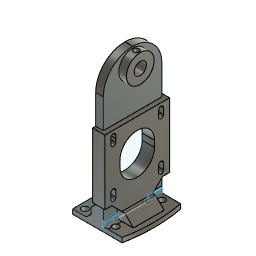
Right handle (Autodesk Fusion 360 design; units mm, degrees)
Autodesk Fusion 360 part; units mm, degrees
note: some values were not read from the file. Set by a fixed rule: which face or edge a step refers to.
sketch "Szkic1" plane through (0, 0, 0) normal (0, 0, 1) x (1, 0, 0)
  circle A0 centre (0, 0) radius 100
  line L0 (66, 19) -> (66, -19)
  line L1 (66, -19) -> (98.1784, -19)
  line L2 (66, 19) -> (98.1784, 19)
  dimension "d1" = 200
  constraint coincident A0.centre origin
  constraint coincident A0 L1.end
  constraint perpendicular L0 L1
  constraint coincident A0 L2.end
  constraint perpendicular L0 L2
  measures "d1" diameter of A0
extrude "Wyciągnięcie proste1" add sketch "Szkic1" along normal blind 3 contours A0 L0 L1 L2 picked at (77.3333, 0)
move_face "Przesuń powierzchnię1" by (-33, 0, 0) 1 faces at (77.3333, 0, 3)
move_body "Przesuń1" bodies 1 to x (1, 0, 0) y (0, 1, 0) z (0, 0, 1) at (-66, 0, 0)
sketch "Szkic2" plane through (0, 0, 3) normal (0, 0, 1) x (-1, 0, 0)
  line L0 (0, 19) -> (-32.1784, 19)
  arc A0 (-32.1784, 19) -> (-32.1784, -19) centre (66, 0) ccw
  line L1 (-32.1784, -19) -> (0, -19)
  line L2 (0, -19) -> (0, 19)
  circle A1 centre (-4, -15) radius 2.1
  circle A2 centre (-24, -15) radius 2.1
  circle A3 centre (-4, 15) radius 2.1
  circle A4 centre (-24, 15) radius 2.1
  dimension "d5" = 4.2
  dimension "d6" = 4.2
  dimension "d7" = 4.2
  dimension "d8" = 4.2
  measures "d5" diameter of A1
  measures "d6" diameter of A2
  measures "d7" diameter of A3
  measures "d8" diameter of A4
extrude "Wyciągnięcie proste2" cut sketch "Szkic2" against normal blind 3 contours A1 | A2 | A3 | A4
sketch "Szkic3" plane through (0, 0, 3) normal (0, 0, 1) x (-1, 0, 0)
  circle A0 centre (-4, 15) radius 2.1
  circle A1 centre (-24, 15) radius 2.1
  circle A2 centre (-4, -15) radius 2.1
  circle A3 centre (-24, -15) radius 2.1
  line L0 (0, 19) -> (-32.1784, 19)
  arc A4 (-32.1784, 19) -> (-32.1784, -19) centre (66, 0) ccw
  line L1 (-32.1784, -19) -> (0, -19)
  line L2 (0, -19) -> (0, 19)
  line L3 (-15, -19) -> (-20, -19)
  line L4 (-20, -19) -> (-20, 19)
  line L5 (-20, 19) -> (-15, 19)
  line L6 (-15, 19) -> (-15, -19)
  constraint horizontal L3
  constraint vertical L4
  constraint horizontal L5
  constraint vertical L6
  constraint coincident L0 L4.end
  constraint coincident L1 L3.start
extrude "Wyciągnięcie proste3" add sketch "Szkic3" along normal blind 72 contours L0 L1 L3 L4 L5 L6
extrude "Wyciągnięcie proste4" add 1 faces at (18.3333, -6.3333, 75) along direction (0, 0, 1) blind 30
extrude "Wyciągnięcie proste5" cut 1 faces at (18.3333, -6.3333, 105) along direction (0, 0, -1) blind 10
sketch "Szkic4" plane through (15, 0, 0) normal (-1, 0, 0) x (0, -1, 0)
  line L0 (19, 95) -> (-19, 95)
  line L1 (-19, 95) -> (-19, 3)
  line L2 (-19, 3) -> (19, 3)
  line L3 (19, 3) -> (19, 95)
  circle A0 centre (0, 85) radius 4
extrude "Wyciągnięcie proste6" cut sketch "Szkic4" against normal blind 5 contours A0
fillet "Zaokrąglenie1" radius 19 2 edges at (17.5, -19, 95) (17.5, 19, 95)
sketch "Szkic5" plane through (20, 0, 0) normal (1, 0, 0) x (0, 1, 0)
  circle A0 centre (0, 85) radius 4
  arc A1 (19, 76) -> (0, 95) centre (0, 76) ccw
  arc A2 (0, 95) -> (-19, 76) centre (0, 76) ccw
  line L0 (-19, 76) -> (-19, 3)
  line L1 (-19, 3) -> (19, 3)
  line L2 (19, 3) -> (19, 76)
  circle A3 centre (0, 85) radius 9
  dimension "d21" = 18
  constraint concentric A0 A3
  measures "d21" diameter of A3
extrude "Wyciągnięcie proste7" add sketch "Szkic5" along normal blind 5 contours A3
sketch "Szkic6" plane through (0, 0, 3) normal (0, 0, 1) x (-1, 0, 0)
  line L0 (-20, -19) -> (-20, 19)
  line L1 (-20, 19) -> (-32.1784, 19)
  arc A0 (-32.1784, 19) -> (-32.1784, -19) centre (66, 0) ccw
  line L2 (-32.1784, -19) -> (-20, -19)
  circle A1 centre (-24, -15) radius 2.1
  circle A2 centre (-24, 15) radius 2.1
  circle A3 through (-20.7, 0, 92.5) (-23.4, 1.5588, 92.5) (-23.4, -1.5588, 92.5)
  dimension "d24" = 3.6
extrude "Wyciągnięcie proste8" cut sketch "Szkic6" against normal blind 8 contours A3 in plane through (0, 0, 95.5) normal (0, 0, 1)
sketch "Szkic7" plane through (0, 0, 0) normal (0, 1, 0) x (1, 0, 0)
  line L0 (20, -35) -> (28, -35)
  line L1 (28, -35) -> (28, -3)
  line L2 (28, -3) -> (20, -3)
  line L3 (20, -3) -> (20, -35)
  line L4 (15, -35) -> (7, -35)
  line L5 (7, -35) -> (7, -3)
  line L6 (7, -3) -> (15, -3)
  line L7 (15, -3) -> (15, -35)
  constraint horizontal L0
  constraint vertical L1
  constraint horizontal L2
  constraint vertical L3
  constraint horizontal L4
  constraint vertical L5
  constraint horizontal L6
  constraint vertical L7
extrude "Wyciągnięcie proste9" add sketch "Szkic7" along normal mid plane 16
extrude "Wyciągnięcie proste10" cut 2 faces at (25.3333, 2.6667, 35) (9.6667, 2.6667, 35) along direction (0, 0, -1) blind 28
sketch "Szkic8" plane through (20, 0, 0) normal (1, 0, 0) x (0, 1, 0)
  line L0 (8, 7) -> (8, 3)
  line L1 (8, 3) -> (19, 3)
  line L2 (19, 3) -> (19, 76)
  arc A0 (19, 76) -> (0, 95) centre (0, 76) ccw
  arc A1 (0, 95) -> (-19, 76) centre (0, 76) ccw
  line L3 (-19, 76) -> (-19, 3)
  line L4 (-19, 3) -> (-8, 3)
  line L5 (-8, 3) -> (-8, 7)
  line L6 (-8, 7) -> (8, 7)
  circle A2 centre (0, 85) radius 9
  line L7 (-8, 7) -> (8, 7)
  line L8 (8, 7) -> (8, 35)
  line L9 (8, 35) -> (-8, 35)
  line L10 (-8, 35) -> (-8, 7)
  constraint horizontal L7
  constraint vertical L8
  constraint horizontal L9
  constraint vertical L10
  constraint coincident L5.end L6.start
extrude "Wyciągnięcie proste11" add sketch "Szkic8" along normal blind 4 and the other way blind 9 contours L6 L7 L8 L9 L10
extrude "Wyciągnięcie proste12" cut 1 faces at (11, 2.6667, 25.6667) along direction (1, 0, 0) blind 1
extrude "Wyciągnięcie proste13" cut 2 faces at (11.3333, -2.6667, 7) (9.6667, -2.6667, 7) along direction (0, 0, -1) blind 2
extrude "Wyciągnięcie proste14" add 2 faces at (14, -8, 5) (13, -8, 25.6667) along direction (0, -1, 0) blind 11
extrude "Wyciągnięcie proste15" add 2 faces at (14, 8, 5) (13, 8, 25.6667) along direction (0, 1, 0) blind 11
extrude "Wyciągnięcie proste16" cut 1 faces at (10.3333, -6.3333, 5) along direction (0, 0, -1) blind 2
extrude "Wyciągnięcie proste17" cut 1 faces at (12, -6.3333, 15) along direction (1, 0, 0) blind 3
fillet "Zaokrąglenie2" radius 6 1 edges at (15, 0, 3)
extrude "Wyciągnięcie proste18" cut 1 faces at (22.6667, 2.6667, 35) along direction (0, 0, -1) blind 20
extrude "Wyciągnięcie proste19" add 1 faces at (28, 2.6667, 5.6667) along direction (1, 0, 0) blind 3
sketch "Szkic9" plane through (15, 0, 0) normal (-1, 0, 0) x (0, -1, 0)
  circle A0 centre (0, 85) radius 4
  line L0 (-19, 9) -> (19, 9)
  line L1 (19, 9) -> (19, 76)
  arc A1 (19, 76) -> (0, 95) centre (0, 76) ccw
  arc A2 (0, 95) -> (-19, 76) centre (0, 76) ccw
  line L2 (-19, 76) -> (-19, 9)
  line L3 (0, 85) -> (0, 36)
  line L4 (15.5, 20.5) -> (-15.5, 51.5) construction
  line L5 (-15.5, 20.5) -> (15.5, 51.5) construction
  circle A3 centre (-15.5, 51.5) radius 1.6
  circle A4 centre (15.5, 51.5) radius 1.6
  circle A5 centre (15.5, 20.5) radius 1.6
  circle A6 centre (-15.5, 20.5) radius 1.6
  point P0 (0, 36)
  dimension "d53" = 31
  dimension "d54" = 31
  dimension "d55" = 3.2
  dimension "d56" = 3.2
  dimension "d57" = 3.2
  dimension "d58" = 3.2
  constraint coincident A0.centre L3.start
  constraint vertical L3
  constraint coincident L4 P0
  constraint coincident L5 P0
  constraint coincident P0 L3.end
  constraint coincident L4.end A3.centre
  constraint coincident L5.end A4.centre
  constraint coincident L4.start A5.centre
  constraint coincident L5.start A6.centre
  measures "d53" distance of L4.end L5.end
  measures "d54" distance of L5.start L4.end
  measures "d55" diameter of A3
  measures "d56" diameter of A4
  measures "d57" diameter of A5
  measures "d58" diameter of A6
extrude "Wyciągnięcie proste20" cut sketch "Szkic9" against normal blind 5 contours A3 | A4 | A5 | A6
sketch "Szkic10" plane through (0, -19, 0) normal (0, -1, 0) x (1, 0, 0)
  arc A0 (9, 3) -> (15, 9) centre (9, 9) ccw
  line L0 (9, 3) -> (0, 3)
  line L1 (0, 3) -> (0, 0)
  line L2 (0, 0) -> (32.1784, 0)
  line L3 (32.1784, 0) -> (32.1784, 3)
  line L4 (32.1784, 3) -> (20, 3)
  line L5 (20, 3) -> (20, 76)
  line L6 (20, 76) -> (15, 76)
  line L7 (15, 76) -> (15, 9)
sketch "Szkic11" plane through (15, 0, 0) normal (-1, 0, 0) x (0, -1, 0)
  circle A0 centre (-15.5, 51.5) radius 1.6
  circle A1 centre (15.5, 51.5) radius 1.6
  circle A2 centre (-15.5, 20.5) radius 1.6
  circle A3 centre (15.5, 20.5) radius 1.6
  circle A4 centre (0, 85) radius 4
  line L0 (-19, 9) -> (19, 9)
  line L1 (19, 9) -> (19, 76)
  arc A5 (19, 76) -> (0, 95) centre (0, 76) ccw
  arc A6 (0, 95) -> (-19, 76) centre (0, 76) ccw
  line L2 (-19, 76) -> (-19, 9)
  line L3 (-15.5, 51.5) -> (15.5, 51.5)
  line L4 (15.5, 51.5) -> (15.5, 20.5)
  line L5 (15.5, 20.5) -> (-15.5, 20.5)
  line L6 (-15.5, 20.5) -> (-15.5, 51.5)
  line L7 (21, 17) -> (-21, 17)
  line L8 (-21, 17) -> (-21, 55)
  line L9 (-21, 55) -> (21, 55)
  line L10 (21, 55) -> (21, 17)
  line L11 (21, 17) -> (-21, 55) construction
  line L12 (-21, 17) -> (21, 55) construction
  line L13 (-19, 55) -> (19, 55)
  line L14 (19, 55) -> (19, 17)
  line L15 (19, 17) -> (-19, 17)
  line L16 (-19, 17) -> (-19, 55)
  point P0 (0, 36)
  dimension "d61" = 42
  constraint horizontal L3
  constraint vertical L4
  constraint horizontal L5
  constraint vertical L6
  constraint coincident A3.centre L4.end
  constraint coincident A0.centre L3.start
  constraint horizontal L7
  constraint perpendicular L7 L8
  constraint parallel L7 L9
  constraint parallel L8 L10
  constraint coincident L11 P0
  constraint coincident L12 P0
  constraint horizontal L13
  constraint vertical L14
  constraint horizontal L15
  constraint vertical L16
  constraint coincident L1 L14.end
  constraint coincident L7 L14.end
  constraint coincident L9 L13.start
  constraint coincident L2 L13.start
  measures "d61" distance of L8.end L9.end
extrude "Wyciągnięcie proste21" add sketch "Szkic11" against normal blind 5 contours L2 L7 L8 L9 L16 | L1 L7 L9 L10 L14
extrude "Wyciągnięcie proste22" cut 1 faces at (22.6667, 2.6667, 15) along direction (0, 0, -1) blind 12
extrude "Wyciągnięcie proste23" cut 1 faces at (31, 2.6667, 5.6667) along direction (-1, 0, 0) blind 9
delete_face "Usuń powierzchnię1" 1 faces at (9.5703, -6.3333, 3.0272)
sketch "Szkic12" plane through (15, 0, 0) normal (-1, 0, 0) x (0, -1, 0)
  circle A0 centre (0, 85) radius 4
  circle A1 centre (15.5, 20.5) radius 1.6
  circle A2 centre (-15.5, 20.5) radius 1.6
  circle A3 centre (15.5, 51.5) radius 1.6
  circle A4 centre (-15.5, 51.5) radius 1.6
  line L0 (-19, 3) -> (19, 3)
  line L1 (19, 3) -> (19, 17)
  line L2 (19, 17) -> (21, 17)
  line L3 (21, 17) -> (21, 55)
  line L4 (21, 55) -> (19, 55)
  line L5 (19, 55) -> (19, 76)
  arc A5 (19, 76) -> (0, 95) centre (0, 76) ccw
  arc A6 (0, 95) -> (-19, 76) centre (0, 76) ccw
  line L6 (-19, 76) -> (-19, 55)
  line L7 (-19, 55) -> (-21, 55)
  line L8 (-21, 55) -> (-21, 17)
  line L9 (-21, 17) -> (-19, 17)
  line L10 (-19, 17) -> (-19, 3)
  line L11 (-19, 3) -> (19, 3)
  line L12 (19, 3) -> (19, 10)
  line L13 (19, 10) -> (-19, 10)
  line L14 (-19, 10) -> (-19, 3)
  constraint horizontal L11
  constraint vertical L12
  constraint horizontal L13
  constraint vertical L14
  constraint midpoint L1 L12.end
  constraint coincident L0.start L10.end
extrude "Wyciągnięcie proste24" add sketch "Szkic12" along normal blind 3 contours L0 L1 L10 L11 L12 L13 L14
sketch "Szkic13" plane through (0, 0, 3) normal (0, 0, 1) x (-1, 0, 0)
  line L0 (-12, 19) -> (-12, -19)
  line L1 (-12, -19) -> (0, -19)
  line L2 (0, -19) -> (0, 19)
  line L3 (0, 19) -> (-12, 19)
  circle A0 centre (-4, -15) radius 2.1
  circle A1 centre (-4, 15) radius 2.1
chamfer "Fazowanie1" distance 3 angle 45 2 edges at (15, 0, 10) (12, 0, 3)
sketch "Szkic14" plane through (20, 0, 0) normal (1, 0, 0) x (0, 1, 0)
  circle A0 centre (15.5, 51.5) radius 1.6
  circle A1 centre (-15.5, 51.5) radius 1.6
  circle A2 centre (15.5, 20.5) radius 1.6
  circle A3 centre (-15.5, 20.5) radius 1.6
  line L0 (-19, 3) -> (19, 3)
  line L1 (19, 3) -> (19, 17)
  line L2 (19, 17) -> (21, 17)
  line L3 (21, 17) -> (21, 55)
  line L4 (21, 55) -> (19, 55)
  line L5 (19, 55) -> (19, 76)
  arc A4 (19, 76) -> (0, 95) centre (0, 76) ccw
  arc A5 (0, 95) -> (-19, 76) centre (0, 76) ccw
  line L6 (-19, 76) -> (-19, 55)
  line L7 (-19, 55) -> (-21, 55)
  line L8 (-21, 55) -> (-21, 17)
  line L9 (-21, 17) -> (-19, 17)
  line L10 (-19, 17) -> (-19, 3)
  circle A6 centre (0, 85) radius 9
  line L11 (-10.169, 3) -> (9.831, 3)
  constraint coincident L0 L11.start
  constraint coincident L0 L11.end
chamfer "Fazowanie2" distance 3 angle 45 1 edges at (20, 0, 3)
sketch "Szkic15" plane through (20, 0, 0) normal (1, 0, 0) x (0, 1, 0)
  line L0 (-19, 6) -> (-10, 6)
  line L1 (-10, 6) -> (-10, 3)
  line L2 (-10, 3) -> (-19, 3)
  line L3 (-19, 3) -> (-19, 6)
  line L4 (19, 6) -> (10, 6)
  line L5 (10, 6) -> (10, 3)
  line L6 (10, 3) -> (19, 3)
  line L7 (19, 3) -> (19, 6)
  constraint horizontal L0
  constraint vertical L1
  constraint horizontal L2
  constraint vertical L3
  constraint horizontal L4
  constraint vertical L5
  constraint horizontal L6
  constraint vertical L7
sketch "Szkic16" plane through (0, -19, 0) normal (0, -1, 0) x (1, 0, 0)
  line L0 (9, 3) -> (0, 3)
  line L1 (0, 3) -> (0, 0)
  line L2 (0, 0) -> (32.1784, 0)
  line L3 (32.1784, 0) -> (32.1784, 3)
  line L4 (32.1784, 3) -> (23, 3)
  line L5 (23, 3) -> (20, 6)
  line L6 (20, 6) -> (20, 17)
  line L7 (20, 17) -> (15, 17)
  line L8 (15, 17) -> (15, 13)
  line L9 (15, 13) -> (12, 10)
  line L10 (12, 10) -> (12, 6)
  line L11 (12, 6) -> (9, 3)
  line L12 (20, 6) -> (20, 3)
  line L13 (20, 3) -> (23, 3)
  line L14 (20, 6) -> (23, 3)
  constraint coincident L5.end L6.start
  constraint parallel L6 L12
  constraint coincident L4.end L5.start
extrude "Wyciągnięcie proste25" cut sketch "Szkic16" against normal blind 9 contours L5 L12 L13 L14
sketch "Szkic17" plane through (0, 19, 0) normal (0, 1, 0) x (-1, 0, 0)
  line L0 (0, 3) -> (-9, 3)
  line L1 (-9, 3) -> (-12, 6)
  line L2 (-12, 6) -> (-12, 10)
  line L3 (-12, 10) -> (-15, 13)
  line L4 (-15, 13) -> (-15, 17)
  line L5 (-15, 17) -> (-20, 17)
  line L6 (-20, 17) -> (-20, 6)
  line L7 (-20, 6) -> (-23, 3)
  line L8 (-23, 3) -> (-32.1784, 3)
  line L9 (-32.1784, 3) -> (-32.1784, 0)
  line L10 (-32.1784, 0) -> (0, 0)
  line L11 (0, 0) -> (0, 3)
  line L12 (-20, 6) -> (-23, 3)
  line L13 (-20, 3) -> (-23, 3)
  line L14 (-20, 6) -> (-20, 3)
  constraint coincident L6.end L7.start
  constraint coincident L7.end L8.start
  constraint parallel L8 L13
  constraint parallel L6 L14
extrude "Wyciągnięcie proste26" cut sketch "Szkic17" against normal blind 9 contours L7 L12 L13 L14
extrude "Wyciągnięcie proste27" cut 1 faces at (21, 10, 4) along direction (0, -1, 0) blind 20
sketch "Szkic18" plane through (12, 0, 0) normal (-1, 0, 0) x (0, -1, 0)
  line L0 (-19, 6) -> (19, 6)
  line L1 (19, 6) -> (19, 10)
  line L2 (19, 10) -> (-19, 10)
  line L3 (-19, 10) -> (-19, 6)
sketch "Szkic19" plane through (20, 0, 0) normal (1, 0, 0) x (0, 1, 0)
  circle A0 centre (0, 10) radius 1.8
  dimension "d79" = 3.6
  measures "d79" diameter of A0
extrude "Wyciągnięcie proste28" cut sketch "Szkic19" against normal blind 5.5
sketch "Szkic20" plane through (0, 19, 0) normal (0, 1, 0) x (-1, 0, 0)
  line L0 (-20, 3) -> (-32.1784, 3)
  line L1 (-32.1784, 3) -> (-32.1784, 0)
  line L2 (-32.1784, 0) -> (0, 0)
  line L3 (0, 0) -> (0, 3)
  line L4 (0, 3) -> (-9, 3)
  line L5 (-9, 3) -> (-12, 6)
  line L6 (-12, 6) -> (-12, 10)
  line L7 (-12, 10) -> (-15, 13)
  line L8 (-15, 13) -> (-15, 17)
  line L9 (-15, 17) -> (-20, 17)
  line L10 (-20, 17) -> (-20, 6)
  line L11 (-20, 6) -> (-20, 3)
  line L12 (-20, 7) -> (-20, 3)
  line L13 (-20, 3) -> (-24, 3)
  line L14 (-24, 3) -> (-20, 7)
  constraint coincident L10 L12.start
  constraint coincident L0.start L11.end
  constraint coincident L0 L13.end
  constraint parallel L0 L13
extrude "Wyciągnięcie proste29" add sketch "Szkic20" against normal blind 29 contours L0 L10 L11 L12 L13 L14
sketch "Szkic21" plane through (0, 19, 0) normal (0, 1, 0) x (-1, 0, 0)
  line L0 (-24, 3) -> (-32.1784, 3)
  line L1 (-32.1784, 3) -> (-32.1784, 0)
  line L2 (-32.1784, 0) -> (0, 0)
  line L3 (0, 0) -> (0, 3)
  line L4 (0, 3) -> (-9, 3)
  line L5 (-9, 3) -> (-12, 6)
  line L6 (-12, 6) -> (-12, 10)
  line L7 (-12, 10) -> (-15, 13)
  line L8 (-15, 13) -> (-15, 17)
  line L9 (-15, 17) -> (-20, 17)
  line L10 (-20, 17) -> (-20, 7)
  line L11 (-20, 7) -> (-24, 3)
  line L12 (-20, 7) -> (-24, 3)
  line L13 (-20, 3) -> (-20, 7)
  line L14 (-20, 3) -> (-24, 3)
  constraint coincident L10.end L11.start
  constraint coincident L0.start L11.end
  constraint parallel L10 L13
  constraint parallel L0 L14
extrude "Wyciągnięcie proste30" cut sketch "Szkic21" against normal blind 9 contours L11 L12 L13 L14
sketch "Szkic23" plane through (15, 0, 0) normal (-1, 0, 0) x (0, -1, 0)
  circle A0 centre (-15.5, 53.5) radius 1.6
  circle A1 centre (-15.5, 18.5) radius 1.6
  circle A2 centre (-15.5, 22.5) radius 1.6
  circle A3 centre (15.5, 18.5) radius 1.6
  circle A4 centre (15.5, 22.5) radius 1.6
  circle A5 centre (15.5, 53.5) radius 1.6
  circle A6 centre (15.5, 49.5) radius 1.6
  circle A7 centre (-15.5, 49.5) radius 1.6
  line L0 (-13.9003, 53.4712) -> (-13.9003, 49.4712)
  line L1 (-17.1, 49.5) -> (-17.1, 53.5)
  line L2 (-13.9003, 53.4712) -> (-13.9003, 49.4712)
  line L3 (13.9003, 49.4712) -> (13.9, 53.4999)
  line L4 (17.0997, 53.4712) -> (17.1, 49.5001)
  line L5 (17.1, 22.5001) -> (17.1, 18.5)
  line L6 (13.9, 18.5) -> (13.9, 22.5)
  line L7 (-13.9003, 22.5287) -> (-13.9, 18.5001)
  line L8 (-17.1, 18.5001) -> (-17.1, 22.5)
  dimension "d98" = 3.2
  dimension "d99" = 3.2
  dimension "d100" = 3.2
  dimension "d101" = 3.2
  dimension "d102" = 3.2
  dimension "d103" = 3.2
  dimension "d104" = 3.2
  dimension "d105" = 3.2
  constraint coincident A0 L0.start
  constraint coincident A7 L0.end
  constraint vertical L0
  constraint coincident A7 L1.start
  constraint coincident A0 L1.end
  constraint tangent A0 L1
  constraint vertical L1
  constraint coincident A6 L3.start
  constraint coincident A5 L3.end
  constraint tangent A5 L3
  constraint coincident A5 L4.start
  constraint coincident A6 L4.end
  constraint tangent A6 L4
  constraint coincident A4 L5.start
  constraint coincident A3 L5.end
  constraint tangent A3 L5
  constraint coincident A3 L6.start
  constraint coincident A4 L6.end
  constraint tangent A4 L6
  constraint vertical L6
  constraint coincident A2 L7.start
  constraint coincident A1 L7.end
  constraint tangent A1 L7
  constraint coincident A1 L8.start
  constraint coincident A2 L8.end
  constraint tangent A2 L8
  measures "d98" diameter of A0
  measures "d99" diameter of A1
  measures "d100" diameter of A2
  measures "d101" diameter of A3
  measures "d102" diameter of A4
  measures "d103" diameter of A5
  measures "d104" diameter of A6
  measures "d105" diameter of A7
extrude "Wyciągnięcie proste31" cut sketch "Szkic23" against normal blind 5 contours A0 | A0 A7 L0 L1 L2 | A7 | A1 | A1 A2 L7 L8 | A2 | A3 | A3 A4 L5 L6 | A4 | A5 | A6 | A5 A6 L3 L4
extrude "Wyciągnięcie proste32" add 1 faces at (16.6667, -19.6667, 55) along direction (0, 0, 1) blind 2
extrude "Wyciągnięcie proste33" add 1 faces at (16.6667, 20.3333, 55) along direction (0, 0, 1) blind 2
extrude "Wyciągnięcie proste34" add 2 faces at (16.6667, -20.3333, 17) (16.6667, 19.6667, 17) along direction (0, 0, -1) blind 2
sketch "Szkic24" plane through (15, 0, 0) normal (-1, 0, 0) x (0, -1, 0)
  line L0 (17.1, 22.5001) -> (17.1, 18.5)
  arc A0 (13.9, 18.5) -> (17.1, 18.5) centre (15.5, 18.5) ccw
  line L1 (13.9, 18.5) -> (13.9, 22.5)
  arc A1 (17.1, 22.5001) -> (13.9, 22.5) centre (15.5, 22.5) ccw
  line L2 (-13.9001, 20.4798) -> (-13.9, 18.5001)
  arc A2 (-17.1, 18.5001) -> (-13.9, 18.5001) centre (-15.5, 18.5) ccw
  line L3 (-17.1, 18.5001) -> (-17.1, 22.5)
  arc A3 (-13.9003, 22.5287) -> (-17.1, 22.5) centre (-15.5, 22.5) ccw
  line L4 (-13.9003, 22.5287) -> (-13.9001, 20.5204)
  arc A4 (-13.9001, 20.4798) -> (-13.9001, 20.5204) centre (-15.5, 20.5) ccw
  line L5 (-13.9003, 53.4712) -> (-13.9003, 51.5287)
  arc A5 (-13.9003, 51.4713) -> (-13.9003, 51.5287) centre (-15.5, 51.5) ccw
  line L6 (-13.9003, 51.4713) -> (-13.9003, 49.4712)
  arc A6 (-17.1, 49.5) -> (-13.9003, 49.4712) centre (-15.5, 49.5) ccw
  line L7 (-17.1, 49.5) -> (-17.1, 53.5)
  arc A7 (-13.9003, 53.4712) -> (-17.1, 53.5) centre (-15.5, 53.5) ccw
  line L8 (-19, 13) -> (19, 13)
  line L9 (19, 13) -> (19, 15)
  line L10 (19, 15) -> (21, 15)
  line L11 (21, 15) -> (21, 57)
  line L12 (21, 57) -> (19, 57)
  line L13 (19, 57) -> (19, 76)
  arc A8 (19, 76) -> (0, 95) centre (0, 76) ccw
  arc A9 (0, 95) -> (-19, 76) centre (0, 76) ccw
  line L14 (-19, 76) -> (-19, 57)
  line L15 (-19, 57) -> (-21, 57)
  line L16 (-21, 57) -> (-21, 15)
  line L17 (-21, 15) -> (-19, 15)
  line L18 (-19, 15) -> (-19, 13)
  line L19 (13.9001, 51.5202) -> (13.9, 53.4999)
  arc A10 (17.0997, 53.4712) -> (13.9, 53.4999) centre (15.5, 53.5) ccw
  line L20 (17.0997, 53.4712) -> (17.0999, 51.5205)
  arc A11 (17.0999, 51.4797) -> (17.0999, 51.5205) centre (15.5, 51.5) ccw
  line L21 (17.0999, 51.4797) -> (17.1, 49.5001)
  arc A12 (13.9003, 49.4712) -> (17.1, 49.5001) centre (15.5, 49.5) ccw
  line L22 (13.9003, 49.4712) -> (13.9001, 51.4796)
  arc A13 (13.9001, 51.5202) -> (13.9001, 51.4796) centre (15.5, 51.5) ccw
  circle A14 centre (0, 85) radius 4
sketch "Szkic25" plane through (20, 0, 0) normal (1, 0, 0) x (0, 1, 0)
  line L0 (-21, 57) -> (21, 57)
  line L1 (21, 57) -> (21, 15)
  line L2 (21, 15) -> (-21, 15)
  line L3 (-21, 15) -> (-21, 57)
  constraint horizontal L0
  constraint vertical L1
  constraint horizontal L2
  constraint vertical L3
extrude "Wyciągnięcie proste35" add sketch "Szkic25" along normal blind 5
extrude "Wyciągnięcie proste36" cut sketch "Szkic24" against normal blind 10 contours L0 A0 L1 A1 | L2 A2 L3 A3 L4 A4 | L5 A5 L6 A6 L7 A7 | L19 A10 L20 A11 L21 A12 L22 A13
extrude "Wyciągnięcie proste37" cut 1 faces at (21.3333, 10, 4.3333) along direction (0, -1, 0) blind 21
sketch "Szkic26" plane through (0, 0, 15) normal (0, 0, -1) x (1, 0, 0)
  line L0 (15, -19) -> (15, -21)
  line L1 (15, -21) -> (25, -21)
  line L2 (25, -21) -> (25, 21)
  line L3 (25, 21) -> (15, 21)
  line L4 (15, 21) -> (15, 19)
  line L5 (15, 19) -> (20, 19)
  line L6 (20, 19) -> (20, -19)
  line L7 (20, -19) -> (15, -19)
  line L8 (20, 10) -> (25, 10)
  line L9 (25, 10) -> (25, -10)
  line L10 (25, -10) -> (20, -10)
  line L11 (20, -10) -> (20, 10)
  constraint horizontal L8
  constraint vertical L9
  constraint horizontal L10
  constraint vertical L11
  constraint coincident L2 L9.end
  constraint coincident L6 L8.start
extrude "Wyciągnięcie proste38" add sketch "Szkic26" along normal blind 12 contours L2 L6 L8 L9 L10 L11
chamfer "Fazowanie3" distance 6.5 angle 45 2 edges at (22.5, -10, 15) (22.5, 10, 15)
chamfer "Fazowanie4" distance 5.5 angle 45 1 edges at (25, 0, 3)
sketch "Szkic27" plane through (15, 0, 0) normal (-1, 0, 0) x (0, -1, 0)
  line L0 (17.1, 22.5001) -> (17.1, 18.5)
  arc A0 (13.9, 18.5) -> (17.1, 18.5) centre (15.5, 18.5) ccw
  line L1 (13.9, 18.5) -> (13.9, 22.5)
  arc A1 (17.1, 22.5001) -> (13.9, 22.5) centre (15.5, 22.5) ccw
  line L2 (-13.9001, 20.4798) -> (-13.9, 18.5001)
  arc A2 (-17.1, 18.5001) -> (-13.9, 18.5001) centre (-15.5, 18.5) ccw
  line L3 (-17.1, 18.5001) -> (-17.1, 22.5)
  arc A3 (-13.9003, 22.5287) -> (-17.1, 22.5) centre (-15.5, 22.5) ccw
  line L4 (-13.9003, 22.5287) -> (-13.9001, 20.5204)
  arc A4 (-13.9001, 20.4798) -> (-13.9001, 20.5204) centre (-15.5, 20.5) ccw
  line L5 (-13.9003, 53.4712) -> (-13.9003, 51.5287)
  arc A5 (-13.9003, 51.4713) -> (-13.9003, 51.5287) centre (-15.5, 51.5) ccw
  line L6 (-13.9003, 51.4713) -> (-13.9003, 49.4712)
  arc A6 (-17.1, 49.5) -> (-13.9003, 49.4712) centre (-15.5, 49.5) ccw
  line L7 (-17.1, 49.5) -> (-17.1, 53.5)
  arc A7 (-13.9003, 53.4712) -> (-17.1, 53.5) centre (-15.5, 53.5) ccw
  line L8 (-19, 13) -> (19, 13)
  line L9 (19, 13) -> (19, 15)
  line L10 (19, 15) -> (21, 15)
  line L11 (21, 15) -> (21, 57)
  line L12 (21, 57) -> (19, 57)
  line L13 (19, 57) -> (19, 76)
  arc A8 (19, 76) -> (0, 95) centre (0, 76) ccw
  arc A9 (0, 95) -> (-19, 76) centre (0, 76) ccw
  line L14 (-19, 76) -> (-19, 57)
  line L15 (-19, 57) -> (-21, 57)
  line L16 (-21, 57) -> (-21, 15)
  line L17 (-21, 15) -> (-19, 15)
  line L18 (-19, 15) -> (-19, 13)
  line L19 (13.9001, 51.5202) -> (13.9, 53.4999)
  arc A10 (17.0997, 53.4712) -> (13.9, 53.4999) centre (15.5, 53.5) ccw
  line L20 (17.0997, 53.4712) -> (17.0999, 51.5205)
  arc A11 (17.0999, 51.4797) -> (17.0999, 51.5205) centre (15.5, 51.5) ccw
  line L21 (17.0999, 51.4797) -> (17.1, 49.5001)
  arc A12 (13.9003, 49.4712) -> (17.1, 49.5001) centre (15.5, 49.5) ccw
  line L22 (13.9003, 49.4712) -> (13.9001, 51.4796)
  arc A13 (13.9001, 51.5202) -> (13.9001, 51.4796) centre (15.5, 51.5) ccw
  circle A14 centre (0, 85) radius 4
  circle A15 centre (-15.5, 53.5) radius 3
  circle A16 centre (15.5, 53.5) radius 3
  circle A17 centre (15.5, 49.5) radius 3
  circle A18 centre (-15.5, 49.5) radius 3
  circle A19 centre (-15.5, 22.5) radius 3
  circle A20 centre (-15.5, 18.5) radius 3
  circle A21 centre (15.5, 18.5) radius 3
  circle A22 centre (15.5, 22.5) radius 3
  line L23 (-12.5001, 53.4712) -> (-12.5, 49.5001)
  line L24 (-18.5, 49.5) -> (-18.5, 53.5)
  line L25 (12.5001, 53.4712) -> (12.5, 49.5001)
  line L26 (18.5, 49.5001) -> (18.5, 53.5)
  line L27 (18.5, 22.5) -> (18.5, 18.5)
  line L28 (12.5, 18.5) -> (12.5, 22.5)
  line L29 (-12.5, 22.5) -> (-12.5, 18.5)
  line L30 (-18.5, 18.5) -> (-18.5, 22.5)
  dimension "d124" = 6
  dimension "d125" = 6
  dimension "d126" = 6
  dimension "d127" = 6
  dimension "d128" = 6
  dimension "d129" = 6
  dimension "d130" = 6
  dimension "d131" = 6
  constraint concentric A7 A15
  constraint concentric A10 A16
  constraint concentric A12 A17
  constraint concentric A6 A18
  constraint concentric A3 A19
  constraint concentric A2 A20
  constraint concentric A0 A21
  constraint concentric A1 A22
  constraint coincident A15 L23.start
  constraint coincident A18 L23.end
  constraint tangent A18 L23
  constraint coincident A18 L24.start
  constraint coincident A15 L24.end
  constraint tangent A15 L24
  constraint parallel L7 L24
  constraint coincident A16 L25.start
  constraint coincident A17 L25.end
  constraint tangent A17 L25
  constraint coincident A17 L26.start
  constraint coincident A16 L26.end
  constraint tangent A16 L26
  constraint coincident A22 L27.start
  constraint coincident A21 L27.end
  constraint tangent A21 L27
  constraint parallel L11 L27
  constraint coincident A21 L28.start
  constraint coincident A22 L28.end
  constraint tangent A22 L28
  constraint parallel L11 L28
  constraint coincident A19 L29.start
  constraint coincident A20 L29.end
  constraint tangent A20 L29
  constraint parallel L28 L29
  constraint coincident A20 L30.start
  constraint coincident A19 L30.end
  constraint tangent A19 L30
  constraint parallel L29 L30
  measures "d124" diameter of A15
  measures "d125" diameter of A16
  measures "d126" diameter of A17
  measures "d127" diameter of A18
  measures "d128" diameter of A19
  measures "d129" diameter of A20
  measures "d130" diameter of A21
  measures "d131" diameter of A22
extrude "Wyciągnięcie proste39" cut sketch "Szkic27" against normal blind 4 contours L0 L1 A1 A21 A22 | L0 A21 A22 | L0 A0 L1 A21 A22 | A21 A22 L27 | L1 A21 A22 | A21 A22 L28 | L2 L4 A4 A19 A20 | L2 A2 L3 A19 A20 | L3 A19 A20 | L3 A3 L4 A19 A20 | A19 A20 L29 | A19 A20 L30 | L5 L7 A7 A15 A18 | L5 A5 L6 A15 A18 | L6 A6 L7 A15 A18 | A15 A18 L23 | L7 A15 A18 | A15 A18 L24 | L19 L22 A13 A16 A17 | L19 A10 L20 A16 A17 | A16 A17 L25 | L21 A12 L22 A16 A17 | A16 A17 L26
extrude "Wyciągnięcie proste40" cut 1 faces at (15, -17.394, 51.4978) along direction (1, 0, 0) blind 4
sketch "Szkic28" plane through (15, 0, 0) normal (-1, 0, 0) x (0, -1, 0)
  circle A0 centre (0, 85) radius 4
  line L0 (-19, 13) -> (19, 13)
  line L1 (19, 13) -> (19, 15)
  line L2 (19, 15) -> (21, 15)
  line L3 (21, 15) -> (21, 57)
  line L4 (21, 57) -> (19, 57)
  line L5 (19, 57) -> (19, 76)
  arc A1 (19, 76) -> (0, 95) centre (0, 76) ccw
  arc A2 (0, 95) -> (-19, 76) centre (0, 76) ccw
  line L6 (-19, 76) -> (-19, 57)
  line L7 (-19, 57) -> (-21, 57)
  line L8 (-21, 57) -> (-21, 15)
  line L9 (-21, 15) -> (-19, 15)
  line L10 (-19, 15) -> (-19, 13)
  line L11 (12.5, 18.5) -> (12.5, 22.5)
  arc A3 (18.5, 22.5) -> (12.5, 22.5) centre (15.5, 22.5) ccw
  line L12 (18.5, 22.5) -> (18.5, 18.5)
  arc A4 (12.5, 18.5) -> (18.5, 18.5) centre (15.5, 18.5) ccw
  arc A5 (18.5, 53.5) -> (12.5001, 53.4712) centre (15.5, 53.5) ccw
  line L13 (18.5, 53.5) -> (18.5, 49.5001)
  arc A6 (12.5, 49.5001) -> (18.5, 49.5001) centre (15.5, 49.5) ccw
  line L14 (12.5, 49.5001) -> (12.5001, 53.4712)
  line L15 (-18.5, 18.5) -> (-18.5, 22.5)
  arc A7 (-12.5, 22.5) -> (-18.5, 22.5) centre (-15.5, 22.5) ccw
  line L16 (-12.5, 22.5) -> (-12.5, 18.5)
  arc A8 (-18.5, 18.5) -> (-12.5, 18.5) centre (-15.5, 18.5) ccw
  line L17 (-18.5, 49.5) -> (-18.5, 53.5)
  arc A9 (-12.5001, 53.4712) -> (-18.5, 53.5) centre (-15.5, 53.5) ccw
  line L18 (-12.5001, 53.4712) -> (-12.5, 49.5001)
  arc A10 (-18.5, 49.5) -> (-12.5, 49.5001) centre (-15.5, 49.5) ccw
  circle A11 centre (0, 34) radius 11.2
  circle A12 centre (0, 38) radius 11.2
  line L19 (-11.2, 38) -> (-11.2, 34)
  line L20 (11.2, 38) -> (11.2, 34)
  dimension "d136" = 22.4
  dimension "d137" = 22.4
  constraint coincident A12 L19.start
  constraint coincident A11 L19.end
  constraint tangent A11 L19
  constraint coincident A11 L20.end
  constraint coincident A12 L20.start
  constraint tangent A11 L20
  measures "d136" diameter of A11
  measures "d137" diameter of A12
extrude "Wyciągnięcie proste41" cut sketch "Szkic28" against normal blind 10 contours A11 A12 | A11 A12 L19 | A11 A12 L20 | A11 A12 | A11 A12
sketch "Szkic29" plane through (15, 0, 0) normal (-1, 0, 0) x (0, -1, 0)
  arc A0 (-11.2, 34) -> (11.2, 34) centre (0, 34) ccw
  line L0 (-11.2, 34) -> (-11.2, 38)
  arc A1 (11.2, 38) -> (-11.2, 38) centre (0, 38) ccw
  line L1 (11.2, 38) -> (11.2, 34)
  circle A2 centre (0, 85) radius 4
  line L2 (-19, 13) -> (19, 13)
  line L3 (19, 13) -> (19, 15)
  line L4 (19, 15) -> (21, 15)
  line L5 (21, 15) -> (21, 57)
  line L6 (21, 57) -> (19, 57)
  line L7 (19, 57) -> (19, 76)
  arc A3 (19, 76) -> (0, 95) centre (0, 76) ccw
  arc A4 (0, 95) -> (-19, 76) centre (0, 76) ccw
  line L8 (-19, 76) -> (-19, 57)
  line L9 (-19, 57) -> (-21, 57)
  line L10 (-21, 57) -> (-21, 15)
  line L11 (-21, 15) -> (-19, 15)
  line L12 (-19, 15) -> (-19, 13)
  line L13 (12.5, 18.5) -> (12.5, 22.5)
  arc A5 (18.5, 22.5) -> (12.5, 22.5) centre (15.5, 22.5) ccw
  line L14 (18.5, 22.5) -> (18.5, 18.5)
  arc A6 (12.5, 18.5) -> (18.5, 18.5) centre (15.5, 18.5) ccw
  arc A7 (18.5, 53.5) -> (12.5001, 53.4712) centre (15.5, 53.5) ccw
  line L15 (18.5, 53.5) -> (18.5, 49.5001)
  arc A8 (12.5, 49.5001) -> (18.5, 49.5001) centre (15.5, 49.5) ccw
  line L16 (12.5, 49.5001) -> (12.5001, 53.4712)
  line L17 (-18.5, 18.5) -> (-18.5, 22.5)
  arc A9 (-12.5, 22.5) -> (-18.5, 22.5) centre (-15.5, 22.5) ccw
  line L18 (-12.5, 22.5) -> (-12.5, 18.5)
  arc A10 (-18.5, 18.5) -> (-12.5, 18.5) centre (-15.5, 18.5) ccw
  line L19 (-18.5, 49.5) -> (-18.5, 53.5)
  arc A11 (-12.5001, 53.4712) -> (-18.5, 53.5) centre (-15.5, 53.5) ccw
  line L20 (-12.5001, 53.4712) -> (-12.5, 49.5001)
  arc A12 (-18.5, 49.5) -> (-12.5, 49.5001) centre (-15.5, 49.5) ccw
  circle A13 centre (0, 85) radius 6
  constraint concentric A2 A13
extrude "Wyciągnięcie proste42" add sketch "Szkic29" along normal blind 2 contours A13
extrude "Wyciągnięcie proste43" cut 2 faces at (25, 0.279, 17.6104) (25, 3.3333, 12.8333) along direction (-1, 0, 0) blind 2
extrude "Wyciągnięcie proste44" cut 1 faces at (13, -5.2961, 84.5032) along direction (1, 0, 0) blind 1
extrude "Wyciągnięcie proste45" add 1 faces at (14, -5.2961, 84.5032) along direction (-1, 0, 0) blind 1
